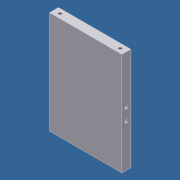
# Autodesk Inventor part: Sides
Saved by Autodesk Inventor 2012 SP1 (Build 160190100, 190)
## iProperties
Created: 2010-12-14
Part Number: Sides
Document SubType Name: Modeling
Designer: berny
Density: 2.71 g/cm^3
Material: Aluminum-6061
Mass: 210.516 g
Surface Area: 207.587 cm^2
Volume: 77.6811 cm^3
Author: berny
Autodesk Inventor part; units mm, degrees
ref_plane "YZ Plane" through (0, 0, 0) normal (1, 0, 0) x (0, 1, 0)
ref_plane "XZ Plane" through (0, 0, 0) normal (0, 1, 0) x (-1, 0, 0)
ref_plane "XY Plane" through (0, 0, 0) normal (0, 0, 1) x (1, 0, 0)
sketch "Sketch1" plane through (0, 0, 0) normal (0, 0, 1) x (1, 0, 0)
  line L0 (0, 0) -> (76.2, 0)
  line L1 (76.2, 0) -> (76.2, 107.95)
  line L2 (76.2, 107.95) -> (0, 107.95)
  line L3 (0, 107.95) -> (0, 0)
  dimension "d0" = 107.95
  dimension "d1" = 76.2
  constraints: 8 end point, 2 parallel, 1 horizontal, 1 perpendicular
  measures "d0" distance of L2.end L0.start
  measures "d1" distance of L0.start L0.end
extrude "Extrusion1" add sketch "Sketch1" along normal blind 9.525
sketch "Sketch2" plane through (76.2, 0, 0) normal (1, 0, 0) x (0, 0, -1)
  line L0 (-9.525, 107.95) -> (-9.525, 0) projected
  line L1 (0, 107.95) -> (-9.525, 107.95) projected
  point P0 (-4.7625, 57.15)
  point P1 (-4.7625, 44.45)
  dimension "d4" = 50.8
  dimension "d5" = 12.7
  dimension "d6" = 4.7625
  constraints: 1 vertical alignment
  measures "d4" distance from line of point (-4.763, 57.15) L1
  measures "d5" distance of point (-4.763, 44.45) point (-4.763, 57.15)
  measures "d6" distance from line of L0 point (-4.763, 57.15)
hole "Hole1" at (76.2, 57.15, 4.7625) at (76.2, 44.45, 4.7625) direction (-1, 0, 0) diameter 3.302 depth 12.7 tip angle 118 thread size "8-32 UNC" class "2B" standard "ANSI Unified Screw Threads"
sketch "Sketch3" plane through (0, 0, 0) normal (0, -1, 0) x (1, 0, 0)
  line L0 (0, 0) -> (0, 9.525) projected
  line L1 (0, 0) -> (76.2, 0) projected
  line L2 (76.2, 0) -> (76.2, 9.525) projected
  point P0 (6.35, 4.7625)
  point P1 (69.85, 4.7625)
  dimension "d14" = 6.35
  dimension "d15" = 6.35
  dimension "d16" = 4.7625
  constraints: 1 horizontal alignment
  measures "d14" distance from line of L2 point (69.85, 4.763)
  measures "d15" distance from line of L0 point (6.35, 4.763)
  measures "d16" distance from line of L1 point (6.35, 4.763)
hole "Hole2" at (6.35, 0, 4.7625) at (69.85, 0, 4.7625) direction (0, 1, 0) diameter 3.302 depth 12.7 tip angle 118 thread size "8-32 UNC" class "2B" standard "ANSI Unified Screw Threads"
sketch "Sketch4" plane through (0, 107.95, 0) normal (0, 1, 0) x (1, 0, 0)
  line L0 (76.2, 0) -> (76.2, -9.525) projected
  line L1 (76.2, 0) -> (0, 0) projected
  line L2 (0, 0) -> (0, -9.525) projected
  point P0 (6.35, -4.7625)
  point P1 (69.85, -4.7625)
  dimension "d24" = 4.7625
  dimension "d25" = 6.35
  dimension "d26" = 6.35
  constraints: 1 horizontal alignment
  measures "d24" distance from line of L1 point (6.35, -4.763)
  measures "d25" distance from line of point (6.35, -4.763) L2
  measures "d26" distance from line of L0 point (69.85, -4.763)
hole "Hole3" at (6.35, 107.95, 4.7625) at (69.85, 107.95, 4.7625) direction (0, -1, 0) diameter 3.302 depth 12.7 tip angle 118 thread size "8-32 UNC" class "2B" standard "ANSI Unified Screw Threads"
body "Solid1"
